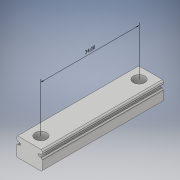
# Autodesk Inventor part: mgn9_carriage_holder
Saved by Autodesk Inventor 2019.4 (Build 234330000, 330)
## iProperties
Created: 2020-10-27
Part Number: mgn9_carriage_holder
Material: Generic
Document SubType Name: Modeling
Designer: PSHUGHAM
Density: 1 g/cm^3
Appearance: Default
Author: PSHUGHAM
Autodesk Inventor part; units mm, degrees
ref_plane "YZ Plane" through (0, 0, 0) normal (1, 0, 0) x (0, 1, 0)
ref_plane "XZ Plane" through (0, 0, 0) normal (0, 1, 0) x (-1, 0, 0)
ref_plane "XY Plane" through (0, 0, 0) normal (0, 0, 1) x (1, 0, 0)
sketch "Sketch1" plane through (0, 0, 0) normal (0, 0, 1) x (1, 0, 0)
  line L0 (8.2, 0) -> (0, 0)
  line L1 (8.6, 0.4) -> (8.2, 0)
  line L2 (8.6, 3.502) -> (8.6, 0.4)
  arc A0 (8.6, 3.502) -> (8.531, 3.6168) centre (8.47, 3.502) ccw
  arc A1 (8.1612, 3.9682) -> (8.531, 3.6168) centre (8.9765, 4.4558) ccw
  arc A2 (8.1612, 3.9682) -> (8.0496, 4.0315) centre (8.0496, 3.9015) ccw
  line L3 (7.7695, 4.0315) -> (8.0496, 4.0315)
  arc A3 (7.7695, 4.8802) -> (7.7695, 4.0315) centre (7.6197, 4.4558) ccw
  line L4 (8.0496, 4.8802) -> (7.7695, 4.8802)
  arc A4 (8.0496, 4.8802) -> (8.1612, 4.9434) centre (8.0496, 5.0102) ccw
  arc A5 (8.531, 5.2949) -> (8.1612, 4.9434) centre (8.9765, 4.4558) ccw
  arc A6 (8.531, 5.2949) -> (8.6, 5.4097) centre (8.47, 5.4097) ccw
  line L5 (8.6, 6.0117) -> (8.6, 5.4097)
  line L6 (8.2, 6.5) -> (8.6, 6.0117)
  line L7 (0, 6.5) -> (8.2, 6.5)
  line L8 (-0.4, 6.0117) -> (0, 6.5)
  line L9 (-0.4, 5.4097) -> (-0.4, 6.0117)
  arc A7 (-0.4, 5.4097) -> (-0.331, 5.2949) centre (-0.27, 5.4097) ccw
  arc A8 (0.0388, 4.9434) -> (-0.331, 5.2949) centre (-0.7765, 4.4558) ccw
  arc A9 (0.0388, 4.9434) -> (0.1504, 4.8802) centre (0.1504, 5.0102) ccw
  line L10 (0.4305, 4.8802) -> (0.1504, 4.8802)
  arc A10 (0.4305, 4.0315) -> (0.4305, 4.8802) centre (0.5803, 4.4558) ccw
  line L11 (0.1504, 4.0315) -> (0.4305, 4.0315)
  arc A11 (0.1504, 4.0315) -> (0.0388, 3.9682) centre (0.1504, 3.9015) ccw
  arc A12 (-0.331, 3.6168) -> (0.0388, 3.9682) centre (-0.7765, 4.4558) ccw
  arc A13 (-0.331, 3.6168) -> (-0.4, 3.502) centre (-0.27, 3.502) ccw
  line L12 (-0.4, 0.4) -> (-0.4, 3.502)
  line L13 (0, 0) -> (-0.4, 0.4)
  point P0 (4.1, 0)
  constraints: 28 end point, 28 point on circle, 14 centre point
extrude "Extrusion1" add sketch "Sketch1" along normal blind 42
sketch "Sketch2" plane through (0, 6.5, 0) normal (0, 1, 0) x (1, 0, 0)
  circle A0 centre (4.1, -4) radius 2
  circle A1 centre (4.1, -38) radius 2
  line L0 (8.2, 0) -> (0, 0) projected
  line L1 (4.1, 0) -> (4.1, -42)
  line L2 (8.2, -42) -> (0, -42) projected
  dimension "d2" = 4
  dimension "d3" = 4
  dimension "d4" = 4
  dimension "d5" = 4
  constraints: 2 centre point, 2 end point, 2 midpoint, 2 point on line
  measures "d2" diameter of A0
  measures "d3" diameter of A1
  measures "d4" distance from line of L0 A0.centre
  measures "d5" distance from line of L2 A1.centre
extrude "Extrusion2" cut sketch "Sketch2" against normal blind 10
body "Solid1"
